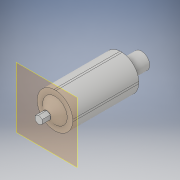
# Autodesk Inventor part: eix bobina
Saved by Autodesk Inventor 2019 (Build 230136000, 136)
## iProperties
Created: 2018-08-16
Part Number: eix bobina
Material: Genérico
Document SubType Name: Modeling
Designer: Albert Garangou Culebras
Density: 1 g/cm^3
Appearance: Valor por defecto
Author: Albert Garangou Culebras
Autodesk Inventor part; units mm, degrees
ref_plane "YZ Plane" through (0, 0, 0) normal (1, 0, 0) x (0, 1, 0)
ref_plane "XZ Plane" through (0, 0, 0) normal (0, 1, 0) x (-1, 0, 0)
ref_plane "XY Plane" through (0, 0, 0) normal (0, 0, 1) x (1, 0, 0)
sketch "Boceto1" plane through (0, 0, 0) normal (0, 0, 1) x (1, 0, 0)
  circle A0 centre (0, 0) radius 21.75
  arc A1 (1.304413, 21.71085) -> (0, 23.055) centre (0, 21.75) ccw
  arc A2 (0, 23.055) -> (-1.304413, 21.71085) centre (0, 21.75) ccw
  line L0 (0, -21.75) -> (0, -23.25)
  arc A3 (0, -23.25) -> (1.499108, -21.698276) centre (0, -21.75) ccw
  arc A4 (-1.499108, -21.698276) -> (0, -23.25) centre (0, -21.75) ccw
  line L1 (21.75, 0) -> (23.055, 0)
  line L2 (-21.75, 0) -> (-23.25, 0)
  arc A5 (-21.698276, 1.499108) -> (-21.698276, -1.499108) centre (-21.75, 0) ccw
  arc A6 (21.71085, -1.304413) -> (21.71085, 1.304413) centre (21.75, 0) ccw
  dimension "d0" = 43.5
  dimension "d2" = 1.5
  dimension "d4" = 1.5
  constraints: 14 point on circle, 6 centre point, 6 coincident, 6 end point, 2 horizontal, 1 vertical, 15 other
  measures "d2" distance of L0.start L0.end
  measures "d4" distance of L2.start L2.end
extrude "Extrusión1" add sketch "Boceto1" along normal blind 81
sketch "Boceto2" plane through (0, 0, 81) normal (0, 0, 1) x (1, 0, 0)
  line L0 (0, 5) -> (4.330127, 2.5)
  line L1 (4.330127, 2.5) -> (4.330127, -2.5)
  line L2 (4.330127, -2.5) -> (0, -5)
  line L3 (0, -5) -> (-4.330127, -2.5)
  line L4 (-4.330127, -2.5) -> (-4.330127, 2.5)
  line L5 (-4.330127, 2.5) -> (0, 5)
  point P0 (0, 0)
  point P1 (0, 0)
  constraints: 12 end point, 1 coincident, 13 other
extrude "Extrusión2" add sketch "Boceto2" along normal blind 20
sketch "Boceto10" plane through (0, 0, 0) normal (0, 0, -1) x (-1, 0, 0)
  circle A0 centre (0, 0) radius 7.5
  dimension "d37" = 15
  constraints: 1 centre point, 1 coincident
  measures "d37" diameter of A0
extrude "Extrusión9" add sketch "Boceto10" along normal blind 25
sketch "Boceto12" plane through (0, 0, 0) normal (0, 0, -1) x (-1, 0, 0)
  circle A0 centre (0, 0) radius 10
  dimension "d40" = 20
  constraints: 1 centre point, 1 coincident
  measures "d40" diameter of A0
extrude "Extrusión10" add sketch "Boceto12" along normal blind 25
sketch "Boceto20" plane through (0, 0, 81) normal (0, 0, 1) x (1, 0, 0)
  circle A0 centre (0, 0) radius 15
  dimension "d61" = 30
  constraints: 1 centre point, 1 coincident
  measures "d61" diameter of A0
ref_plane "Plano de trabajo1" through (0, 0, 91) normal (0, 0, 1) x (1, 0, 0)
sketch "Boceto21" plane through (0, 0, 91) normal (0, 0, 1) x (1, 0, 0)
  line L0 (4.330127, 2.5) -> (4.330127, -2.5)
  circle A0 centre (0, 0) radius 5
  constraints: 1 coincident, 3 other
sketch "Boceto20 outline for Solevación1" plane through (0, 0, 81) normal (0, 0, 1) x (1, 0, 0)
  circle A0 centre (0, 0) radius 15
sketch "Boceto21 outline for Solevación1" plane through (0, 0, 91) normal (0, 0, 1) x (1, 0, 0)
  circle A0 centre (0, 0) radius 5
loft "Solevación1" add profiles "Boceto20 outline for Solevación1", "Boceto21 outline for Solevación1"
sketch "Boceto22" plane through (0, 0, 81) normal (0, 0, 1) x (1, 0, 0)
  arc A0 (1.304413, 21.71085) -> (-1.304413, 21.71085) centre (0, 21.75) ccw
  arc A1 (1.304413, 21.71085) -> (-1.304413, 21.71085) centre (0, 21.749554) ccw
  arc A2 (21.71085, -1.304413) -> (21.71085, 1.304413) centre (21.75, 0) ccw
  arc A3 (21.71085, -1.304413) -> (21.71085, 1.304413) centre (21.749554, 0) ccw
  arc A4 (-1.499108, -21.698276) -> (1.499108, -21.698276) centre (0, -21.75) ccw
  arc A5 (-1.499108, -21.698276) -> (1.499108, -21.698276) centre (0, -21.749411) ccw
  arc A6 (-21.698276, 1.499108) -> (-21.698276, -1.499108) centre (-21.75, 0) ccw
  arc A7 (-21.685394, 1.49099) -> (-21.698276, -1.499108) centre (-21.753079, -0.003795) ccw
  arc A8 (-21.698276, 1.499108) -> (-21.698276, -1.499108) centre (-1.222086, 0) ccw
  arc A9 (1.304413, 21.71085) -> (-1.304413, 21.71085) centre (0, -0.250446) ccw
  arc A10 (21.71085, -1.304413) -> (21.71085, 1.304413) centre (-0.250446, 0) ccw
  arc A11 (-1.499108, -21.698276) -> (1.499108, -21.698276) centre (0, 0.250589) ccw
  point P0 (0, 0)
  constraints: 20 point on circle, 8 centre point
sketch "Boceto22 outline for Extrusión16" plane through (0, 0, 81) normal (0, 0, 1) x (1, 0, 0)
  arc A0 (-1.304413, 21.71085) -> (1.304413, 21.71085) centre (0, -0.250446) cw
  arc A1 (1.304413, 21.71085) -> (-1.304413, 21.71085) centre (0, 21.75) ccw
  arc A2 (21.71085, 1.304413) -> (21.71085, -1.304413) centre (-0.250446, 0) cw
  arc A3 (21.71085, -1.304413) -> (21.71085, 1.304413) centre (21.75, 0) ccw
  arc A4 (-21.698276, -1.499108) -> (-21.698276, 1.499108) centre (-1.222086, 0) cw
  arc A5 (-21.698276, 1.499108) -> (-21.698276, -1.499108) centre (-21.75, 0) ccw
  arc A6 (1.499108, -21.698276) -> (-1.499108, -21.698276) centre (0, 0.250589) cw
  arc A7 (-1.499108, -21.698276) -> (1.499108, -21.698276) centre (0, -21.75) ccw
extrude "Extrusión16" cut sketch "Boceto22 outline for Extrusión16" against normal blind 211
